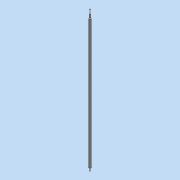
# Autodesk Inventor part: Śruba trapezowa fi10mm
Saved by Autodesk Inventor 2018 (Build 220112000, 112)
## iProperties
Created: 2019-01-23
Part Number: Śruba trapezowa fi10mm
Material: Ogólny
Document SubType Name: Modeling
Designer: Dawid
Density: 1 g/cm^3
Appearance: Domyślna
Author: Dawid
Autodesk Inventor part; units mm, degrees
ref_plane "YZ Plane" through (0, 0, 0) normal (1, 0, 0) x (0, 1, 0)
ref_plane "XZ Plane" through (0, 0, 0) normal (0, 1, 0) x (-1, 0, 0)
ref_plane "XY Plane" through (0, 0, 0) normal (0, 0, 1) x (1, 0, 0)
sketch "Szkic1" plane through (0, 0, 0) normal (0, 0, 1) x (1, 0, 0)
  circle A0 centre (0, 0) radius 8
  dimension "d0" = 16
  constraints: 1 centre point, 1 coincident
  measures "d0" diameter of A0
extrude "Wyciągnięcie proste2" add sketch "Szkic1" along normal blind 1000
sketch "Szkic2" plane through (0, 0, 1000) normal (0, 0, 1) x (1, 0, 0)
  circle A0 centre (0, 0) radius 4
  circle A1 centre (0, 0) radius 8 projected
  dimension "d7" = 8
  constraints: 1 centre point, 1 coincident
  measures "d7" diameter of A0
extrude "Wyciągnięcie proste3" cut sketch "Szkic2" against normal blind 30
sketch "Szkic3" plane through (0, 0, 970) normal (0, 0, 1) x (1, 0, 0)
  circle A0 centre (0, 0) radius 8 projected
  circle A1 centre (0, 0) radius 5
  dimension "d10" = 10
  constraints: 1 centre point, 1 coincident
  measures "d10" diameter of A1
extrude "Wyciągnięcie proste4" cut sketch "Szkic3" against normal blind 30
sketch "Szkic4" plane through (0, 0, 970) normal (0, 0, 1) x (1, 0, 0)
  circle A0 centre (0, 0) radius 5 projected
  circle A1 centre (0, 0) radius 4.98
  dimension "d13" = 9.96
  constraints: 1 centre point, 1 coincident
  measures "d13" diameter of A1
extrude "Wyciągnięcie proste5" cut sketch "Szkic4" against normal blind 20
thread "Gwint2" size "M10x1.5" class "6g" standard "ANSI Metric M Profile" full length
sketch "Szkic5" plane through (0, 0, 0) normal (0, 0, -1) x (-1, 0, 0)
  circle A0 centre (0, 0) radius 5
  circle A1 centre (0, 0) radius 8 projected
  dimension "d18" = 10
  constraints: 1 centre point, 1 coincident
  measures "d18" diameter of A0
extrude "Wyciągnięcie proste6" cut sketch "Szkic5" against normal blind 20
thread "Gwint3" size "TR16x4" class "7e" standard "ISO Metric Trapezoidal Threads" full length
sketch "Szkic6" plane through (0, 0, 940) normal (0, 0, 1) x (1, 0, 0)
  circle A0 centre (0, 0) radius 5 projected
  circle A1 centre (0, 0) radius 8 projected
extrude "Wyciągnięcie proste7" cut sketch "Szkic6" against normal blind 14
sketch "Szkic7" plane through (0, 0, 950) normal (0, 0, 1) x (1, 0, 0)
  circle A0 centre (0, 0) radius 4.98 projected
  circle A1 centre (0, 0) radius 5 projected
extrude "Wyciągnięcie proste8" cut sketch "Szkic7" against normal blind 15
sketch "Szkic8" plane through (0, 0, 970) normal (0, 0, 1) x (1, 0, 0)
  circle A0 centre (0, 0) radius 4.98 projected
  circle A1 centre (0, 0) radius 4 projected
extrude "Wyciągnięcie proste9" cut sketch "Szkic8" against normal blind 15
sketch "Szkic9" plane through (0, 0, 1000) normal (0, 0, 1) x (1, 0, 0)
  circle A0 centre (0, 0) radius 4 projected
extrude "Wyciągnięcie proste10" cut sketch "Szkic9" against normal blind 15.9
